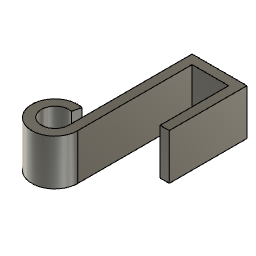
WireClamp (Autodesk Fusion 360 design; units mm, degrees)
Autodesk Fusion 360 part; units mm, degrees
sketch "Skizze1" plane through (0, 0, 0) normal (0, 0, 1) x (1, 0, 0)
  line L0 (8, 0) -> (8, 15)
  line L1 (8, 15) -> (0, 15)
  line L2 (0, 15) -> (0, -10)
  line L3 (8, 0) -> (10, 0)
  line L4 (10, 0) -> (10, 17)
  line L5 (10, 17) -> (-2, 17)
  line L6 (-2, 17) -> (-2, -10)
  line L7 (-2, -10) -> (0, -10)
  circle A0 centre (-4.9997, -10.052) radius 5
  circle A1 centre (-4.9999, -9.9716) radius 3
  line L8 (-3.9109, -5.172) -> (-4.9999, -9.9716)
  dimension "d2" = 8
  dimension "d3" = 15
  dimension "d4" = 25
  dimension "d5" = 2
  dimension "d6" = 2
  dimension "d7" = 2
  dimension "d8" = 10
  dimension "d9" = 6
  constraint vertical L0
  constraint perpendicular L0 L1
  constraint perpendicular L1 L2
  constraint coincident origin L2
  constraint perpendicular L0 L3
  constraint perpendicular L3 L4
  constraint perpendicular L4 L5
  constraint perpendicular L3 L6
  constraint parallel L5 L7
  constraint coincident origin L3
  constraint coincident L2.end A0
  constraint coincident L6.end A1
  constraint coincident A0 L8.start
  constraint coincident A1.centre L8.end
  measures "d2" distance of L0.end L1.end
  measures "d3" distance of L0.start L0.end
  measures "d4" distance of L1.end L2.end
  measures "d5" distance of L0 L4
  measures "d6" distance of L1 L5
  measures "d7" distance of L2 L6
  measures "d8" diameter of A0
  measures "d9" diameter of A1
extrude "Extrusion1" add sketch "Skizze1" along normal blind 10 contours L0 L1 L2 L3 L4 L5 L6 A0 | L7 A0 A1 L8 | L6 L7 A0 A1
equation "d6 = d5"
equation "d7 = d5"
named bodies: "WireClamp"
